Autodesk Fusion 360 part; units mm, degrees
(part 17 of 20)
  spline S293 degree 3 poles (21.9659, -337.034) (21.9695, -336.7657) (21.976, -336.2825) (22.0953, -335.8147) (22.1484, -335.6066) knots 0 0 0 0 0.080152 0.144341 0.144341 0.144341 0.144341
  spline S294 degree 3 poles (22.1484, -335.6066) (22.213, -335.4398) (22.3355, -335.1233) (22.5766, -334.8853) (22.6906, -334.7727) knots 0 0 0 0 0.052977 0.10048 0.10048 0.10048 0.10048
  spline S295 degree 3 poles (22.6906, -334.7727) (22.822, -334.6872) (23.0969, -334.5083) (23.4249, -334.4893) (23.5961, -334.4794) knots 0 0 0 0 0.046203 0.096661 0.096661 0.096661 0.096661
  spline S296 degree 3 poles (23.5961, -334.4794) (23.7239, -334.485) (23.9694, -334.4957) (24.1943, -334.5941) (24.3022, -334.6414) knots 0 0 0 0 0.037989 0.072993 0.072993 0.072993 0.072993
  spline S297 degree 3 poles (24.3022, -334.6414) (24.3994, -334.7021) (24.5968, -334.8252) (24.7339, -335.0132) (24.8035, -335.1086) knots 0 0 0 0 0.034048 0.069103 0.069103 0.069103 0.069103
  spline S298 degree 3 poles (24.8035, -335.1086) (24.8668, -335.2196) (25.0009, -335.4545) (25.0749, -335.7148) (25.1139, -335.8521) knots 0 0 0 0 0.038176 0.080832 0.080832 0.080832 0.080832
  spline S299 degree 3 poles (25.1139, -335.8521) (25.1466, -336.0232) (25.2212, -336.4133) (25.2246, -336.8107) (25.2265, -337.0339) knots 0 0 0 0 0.052146 0.118926 0.118926 0.118926 0.118926
  spline S300 degree 3 poles (25.2265, -337.0339) (25.2229, -337.3005) (25.2163, -337.7813) (25.0983, -338.247) (25.0458, -338.4545) knots 0 0 0 0 0.079639 0.143634 0.143634 0.143634 0.143634
  spline S301 degree 3 poles (25.0458, -338.4545) (24.9816, -338.6214) (24.8598, -338.9384) (24.6191, -339.1771) (24.5052, -339.2901) knots 0 0 0 0 0.052961 0.100531 0.100531 0.100531 0.100531
  spline S302 degree 3 poles (24.5052, -339.2901) (24.3736, -339.3761) (24.0979, -339.5562) (23.7684, -339.5752) (23.5963, -339.5851) knots 0 0 0 0 0.046339 0.097057 0.097057 0.097057 0.097057
  spline S303 degree 3 poles (23.5963, -339.5851) (23.37, -339.5658) (22.9288, -339.5281) (22.6139, -339.2179) (22.4605, -339.0667) knots 0 0 0 0 0.065835 0.128409 0.128409 0.128409 0.128409
  spline S304 degree 3 poles (22.4605, -339.0667) (22.3171, -338.7986) (21.9794, -338.1676) (21.9709, -337.4479) (21.9659, -337.034) knots 0 0 0 0 0.090022 0.211899 0.211899 0.211899 0.211899
  line L400 (28.3848, -338.173) -> (28.9885, -338.2514)
  spline S305 degree 3 poles (28.9885, -338.2514) (28.9458, -338.4453) (28.864, -338.8171) (28.6056, -339.0954) (28.482, -339.2286) knots 0 0 0 0 0.058356 0.111856 0.111856 0.111856 0.111856
  spline S306 degree 3 poles (28.482, -339.2286) (28.3359, -339.3315) (28.0358, -339.543) (27.6692, -339.5685) (27.481, -339.5816) knots 0 0 0 0 0.052559 0.107965 0.107965 0.107965 0.107965
  spline S307 degree 3 poles (27.481, -339.5816) (27.2479, -339.5641) (26.7963, -339.5302) (26.4521, -339.2373) (26.2856, -339.0956) knots 0 0 0 0 0.068154 0.132052 0.132052 0.132052 0.132052
  spline S308 degree 3 poles (26.2856, -339.0956) (26.154, -338.9049) (25.8661, -338.4875) (25.8451, -337.9787) (25.8336, -337.7024) knots 0 0 0 0 0.068157 0.149141 0.149141 0.149141 0.149141
  spline S309 degree 3 poles (25.8336, -337.7024) (25.8399, -337.5171) (25.8519, -337.1646) (25.9713, -336.8331) (26.028, -336.6758) knots 0 0 0 0 0.055211 0.105055 0.105055 0.105055 0.105055
  spline S310 degree 3 poles (26.028, -336.6758) (26.1002, -336.5389) (26.2424, -336.2693) (26.4952, -336.0994) (26.6197, -336.0158) knots 0 0 0 0 0.04564 0.089884 0.089884 0.089884 0.089884
  spline S311 degree 3 poles (26.6197, -336.0158) (26.7556, -335.9516) (27.0295, -335.8223) (27.332, -335.8047) (27.4843, -335.7958) knots 0 0 0 0 0.044643 0.089956 0.089956 0.089956 0.089956
  spline S312 degree 3 poles (27.4843, -335.7958) (27.668, -335.8052) (28.0159, -335.8229) (28.3105, -336.0072) (28.4495, -336.0942) knots 0 0 0 0 0.054149 0.102527 0.102527 0.102527 0.102527
  spline S313 degree 3 poles (28.4495, -336.0942) (28.564, -336.2077) (28.8031, -336.4447) (28.8868, -336.7715) (28.9305, -336.9417) knots 0 0 0 0 0.047449 0.099081 0.099081 0.099081 0.099081
  line L401 (28.9305, -336.9417) -> (28.3336, -337.0338)
  spline S314 degree 3 poles (28.3336, -337.0338) (28.3027, -336.9224) (28.2453, -336.715) (28.0993, -336.5576) (28.0317, -336.4847) knots 0 0 0 0 0.034086 0.063475 0.063475 0.063475 0.063475
  spline S315 degree 3 poles (28.0317, -336.4847) (27.9547, -336.431) (27.7974, -336.3213) (27.606, -336.3076) (27.5082, -336.3006) knots 0 0 0 0 0.027619 0.056426 0.056426 0.056426 0.056426
  spline S316 degree 3 poles (27.5082, -336.3006) (27.3615, -336.3136) (27.0724, -336.3393) (26.8594, -336.5361) (26.7545, -336.6331) knots 0 0 0 0 0.04285 0.084486 0.084486 0.084486 0.084486
  spline S317 degree 3 poles (26.7545, -336.6331) (26.6703, -336.7727) (26.4764, -337.0942) (26.4688, -337.4717) (26.4646, -337.6853) knots 0 0 0 0 0.048123 0.11083 0.11083 0.11083 0.11083
  spline S318 degree 3 poles (26.4646, -337.6853) (26.4682, -337.9011) (26.4745, -338.2798) (26.6631, -338.6058) (26.7443, -338.746) knots 0 0 0 0 0.063398 0.111295 0.111295 0.111295 0.111295
  spline S319 degree 3 poles (26.7443, -338.746) (26.8454, -338.8425) (27.05, -339.0376) (27.3317, -339.0637) (27.4742, -339.0768) knots 0 0 0 0 0.040675 0.082263 0.082263 0.082263 0.082263
  spline S320 degree 3 poles (27.4742, -339.0768) (27.5886, -339.0686) (27.8114, -339.0526) (27.9906, -338.9198) (28.0778, -338.8551) knots 0 0 0 0 0.033628 0.065508 0.065508 0.065508 0.065508
  spline S321 degree 3 poles (28.0778, -338.8551) (28.1519, -338.7651) (28.3154, -338.5665) (28.3602, -338.3121) (28.3848, -338.173) knots 0 0 0 0 0.034396 0.07593 0.07593 0.07593 0.07593
  line L402 (21.9646, -288.1562) -> (22.6093, -288.1016)
  spline S322 degree 3 poles (22.6093, -288.1016) (22.637, -288.2449) (22.6882, -288.5098) (22.862, -288.715) (22.9418, -288.8093) knots 0 0 0 0 0.042908 0.079365 0.079365 0.079365 0.079365
  spline S323 degree 3 poles (22.9418, -288.8093) (23.034, -288.8785) (23.2206, -289.0184) (23.4533, -289.037) (23.5711, -289.0464) knots 0 0 0 0 0.033826 0.068485 0.068485 0.068485 0.068485
  spline S324 degree 3 poles (23.5711, -289.0464) (23.7135, -289.0321) (24.0003, -289.0033) (24.2139, -288.8096) (24.3214, -288.7121) knots 0 0 0 0 0.041772 0.0841 0.0841 0.0841 0.0841
  spline S325 degree 3 poles (24.3214, -288.7121) (24.4109, -288.5871) (24.6001, -288.3226) (24.6186, -287.997) (24.6284, -287.8254) knots 0 0 0 0 0.045186 0.095569 0.095569 0.095569 0.095569
  spline S326 degree 3 poles (24.6284, -287.8254) (24.6193, -287.663) (24.6022, -287.3567) (24.4193, -287.1117) (24.3333, -286.9966) knots 0 0 0 0 0.047557 0.089725 0.089725 0.089725 0.089725
  spline S327 degree 3 poles (24.3333, -286.9966) (24.2248, -286.9081) (24.0003, -286.7248) (23.7106, -286.7039) (23.5608, -286.693) knots 0 0 0 0 0.040971 0.08482 0.08482 0.08482 0.08482
  spline S328 degree 3 poles (23.5608, -286.693) (23.4652, -286.6982) (23.2778, -286.7082) (23.1083, -286.7885) (23.0253, -286.8277) knots 0 0 0 0 0.028423 0.055689 0.055689 0.055689 0.055689
  spline S329 degree 3 poles (23.0253, -286.8277) (22.9505, -286.8753) (22.8036, -286.9685) (22.7007, -287.1086) (22.6502, -287.1773) knots 0 0 0 0 0.026342 0.051681 0.051681 0.051681 0.051681
  line L403 (22.6502, -287.1773) -> (22.0738, -287.1023)
  line L404 (22.0738, -287.1023) -> (22.5581, -284.5341)
  line L405 (22.5581, -284.5341) -> (25.0444, -284.5341)
  line L406 (25.0444, -284.5341) -> (25.0444, -285.1207)
  line L407 (25.0444, -285.1207) -> (23.0492, -285.1207)
  line L408 (23.0492, -285.1207) -> (22.7798, -286.4645)
  spline S330 degree 3 poles (22.7798, -286.4645) (22.9293, -286.373) (23.2201, -286.195) (23.5596, -286.1652) (23.7245, -286.1507) knots 0 0 0 0 0.051785 0.100763 0.100763 0.100763 0.100763
  spline S331 degree 3 poles (23.7245, -286.1507) (23.9338, -286.1691) (24.3494, -286.2056) (24.6702, -286.472) (24.8296, -286.6043) knots 0 0 0 0 0.061424 0.122014 0.122014 0.122014 0.122014
  spline S332 degree 3 poles (24.8296, -286.6043) (24.9609, -286.7698) (25.2317, -287.1111) (25.2634, -287.5465) (25.2798, -287.7708) knots 0 0 0 0 0.061868 0.12764 0.12764 0.12764 0.12764
  spline S333 degree 3 poles (25.2798, -287.7708) (25.2646, -287.9877) (25.2347, -288.4136) (24.9995, -288.7695) (24.8842, -288.944) knots 0 0 0 0 0.064036 0.125703 0.125703 0.125703 0.125703
  spline S334 degree 3 poles (24.8842, -288.944) (24.7064, -289.1211) (24.3434, -289.4828) (23.8321, -289.528) (23.5711, -289.5511) knots 0 0 0 0 0.072854 0.148822 0.148822 0.148822 0.148822
  spline S335 degree 3 poles (23.5711, -289.5511) (23.3578, -289.5384) (22.9503, -289.514) (22.6166, -289.2805) (22.4575, -289.1691) knots 0 0 0 0 0.062678 0.119794 0.119794 0.119794 0.119794
  spline S336 degree 3 poles (22.4575, -289.1691) (22.3288, -289.0288) (22.0646, -288.7404) (21.9985, -288.3543) (21.9646, -288.1562) knots 0 0 0 0 0.055877 0.114795 0.114795 0.114795 0.114795
  line L409 (28.3835, -288.1391) -> (28.9872, -288.2176)
  spline S337 degree 3 poles (28.9872, -288.2176) (28.9445, -288.4115) (28.8627, -288.7832) (28.6043, -289.0616) (28.4807, -289.1947) knots 0 0 0 0 0.058356 0.111856 0.111856 0.111856 0.111856
  spline S338 degree 3 poles (28.4807, -289.1947) (28.3346, -289.2977) (28.0345, -289.5091) (27.6678, -289.5346) (27.4797, -289.5477) knots 0 0 0 0 0.052559 0.107965 0.107965 0.107965 0.107965
  spline S339 degree 3 poles (27.4797, -289.5477) (27.2466, -289.5302) (26.795, -289.4963) (26.4508, -289.2034) (26.2842, -289.0617) knots 0 0 0 0 0.068154 0.132052 0.132052 0.132052 0.132052
  spline S340 degree 3 poles (26.2842, -289.0617) (26.1527, -288.871) (25.8648, -288.4536) (25.8437, -287.9448) (25.8323, -287.6685) knots 0 0 0 0 0.068157 0.149141 0.149141 0.149141 0.149141
  spline S341 degree 3 poles (25.8323, -287.6685) (25.8386, -287.4832) (25.8506, -287.1307) (25.9701, -286.7992) (26.0267, -286.6419) knots 0 0 0 0 0.055211 0.105055 0.105055 0.105055 0.105055
  spline S342 degree 3 poles (26.0267, -286.6419) (26.0989, -286.505) (26.2411, -286.2353) (26.494, -286.0655) (26.6185, -285.9819) knots 0 0 0 0 0.04564 0.089884 0.089884 0.089884 0.089884
  spline S343 degree 3 poles (26.6185, -285.9819) (26.7544, -285.9177) (27.0283, -285.7884) (27.3307, -285.7708) (27.4831, -285.7619) knots 0 0 0 0 0.044643 0.089955 0.089955 0.089955 0.089955
  spline S344 degree 3 poles (27.4831, -285.7619) (27.6668, -285.7713) (28.0147, -285.7891) (28.3093, -285.9734) (28.4483, -286.0603) knots 0 0 0 0 0.054149 0.102527 0.102527 0.102527 0.102527
  spline S345 degree 3 poles (28.4483, -286.0603) (28.5627, -286.1738) (28.8018, -286.4109) (28.8855, -286.7376) (28.9292, -286.9079) knots 0 0 0 0 0.047449 0.099081 0.099081 0.099081 0.099081
  line L410 (28.9292, -286.9079) -> (28.3323, -287)
  spline S346 degree 3 poles (28.3323, -287) (28.3014, -286.8886) (28.244, -286.6811) (28.098, -286.5237) (28.0305, -286.4509) knots 0 0 0 0 0.034086 0.063475 0.063475 0.063475 0.063475
  spline S347 degree 3 poles (28.0305, -286.4509) (27.9535, -286.3971) (27.7962, -286.2874) (27.6047, -286.2737) (27.5069, -286.2667) knots 0 0 0 0 0.027619 0.056426 0.056426 0.056426 0.056426
  spline S348 degree 3 poles (27.5069, -286.2667) (27.3603, -286.2797) (27.0711, -286.3054) (26.8581, -286.5022) (26.7532, -286.5992) knots 0 0 0 0 0.04285 0.084486 0.084486 0.084486 0.084486
  spline S349 degree 3 poles (26.7532, -286.5992) (26.669, -286.7388) (26.4751, -287.0603) (26.4676, -287.4378) (26.4633, -287.6514) knots 0 0 0 0 0.048123 0.11083 0.11083 0.11083 0.11083
  spline S350 degree 3 poles (26.4633, -287.6514) (26.4669, -287.8672) (26.4732, -288.2459) (26.6618, -288.5718) (26.743, -288.7121) knots 0 0 0 0 0.063398 0.111295 0.111295 0.111295 0.111295
  spline S351 degree 3 poles (26.743, -288.7121) (26.8441, -288.8086) (27.0487, -289.0037) (27.3304, -289.0298) (27.4728, -289.0429) knots 0 0 0 0 0.040675 0.082263 0.082263 0.082263 0.082263
  spline S352 degree 3 poles (27.4728, -289.0429) (27.5872, -289.0347) (27.8101, -289.0187) (27.9893, -288.8859) (28.0765, -288.8213) knots 0 0 0 0 0.033628 0.065508 0.065508 0.065508 0.065508
  spline S353 degree 3 poles (28.0765, -288.8213) (28.1506, -288.7313) (28.314, -288.5326) (28.3589, -288.2783) (28.3835, -288.1391) knots 0 0 0 0 0.034395 0.07593 0.07593 0.07593 0.07593
  spline S354 degree 3 poles (21.9779, -237.0342) (21.9815, -236.7658) (21.988, -236.2826) (22.1073, -235.8148) (22.1603, -235.6068) knots 0 0 0 0 0.080152 0.144341 0.144341 0.144341 0.144341
  spline S355 degree 3 poles (22.1603, -235.6068) (22.225, -235.4399) (22.3475, -235.1235) (22.5886, -234.8854) (22.7026, -234.7729) knots 0 0 0 0 0.052977 0.10048 0.10048 0.10048 0.10048
  spline S356 degree 3 poles (22.7026, -234.7729) (22.834, -234.6874) (23.1089, -234.5085) (23.4369, -234.4895) (23.6082, -234.4796) knots 0 0 0 0 0.046203 0.096661 0.096661 0.096661 0.096661
  spline S357 degree 3 poles (23.6082, -234.4796) (23.7359, -234.4852) (23.9814, -234.4959) (24.2063, -234.5944) (24.3142, -234.6416) knots 0 0 0 0 0.037989 0.072993 0.072993 0.072993 0.072993
  spline S358 degree 3 poles (24.3142, -234.6416) (24.4114, -234.7023) (24.6088, -234.8255) (24.7459, -235.0135) (24.8155, -235.1089) knots 0 0 0 0 0.034048 0.069103 0.069103 0.069103 0.069103
  spline S359 degree 3 poles (24.8155, -235.1089) (24.8788, -235.2198) (25.0128, -235.4547) (25.0868, -235.715) (25.1259, -235.8524) knots 0 0 0 0 0.038176 0.080832 0.080832 0.080832 0.080832
  spline S360 degree 3 poles (25.1259, -235.8524) (25.1586, -236.0234) (25.2332, -236.4136) (25.2365, -236.811) (25.2384, -237.0342) knots 0 0 0 0 0.052146 0.118926 0.118926 0.118926 0.118926
  spline S361 degree 3 poles (25.2384, -237.0342) (25.2348, -237.3008) (25.2282, -237.7816) (25.1102, -238.2472) (25.0577, -238.4547) knots 0 0 0 0 0.079639 0.143634 0.143634 0.143634 0.143634
  spline S362 degree 3 poles (25.0577, -238.4547) (24.9935, -238.6217) (24.8716, -238.9386) (24.631, -239.1773) (24.5171, -239.2903) knots 0 0 0 0 0.052961 0.100531 0.100531 0.100531 0.100531
  spline S363 degree 3 poles (24.5171, -239.2903) (24.3854, -239.3763) (24.1097, -239.5564) (23.7803, -239.5754) (23.6081, -239.5853) knots 0 0 0 0 0.046338 0.097057 0.097057 0.097057 0.097057
  spline S364 degree 3 poles (23.6081, -239.5853) (23.3819, -239.566) (22.9406, -239.5283) (22.6258, -239.2181) (22.4724, -239.0669) knots 0 0 0 0 0.065835 0.128409 0.128409 0.128409 0.128409
  spline S365 degree 3 poles (22.4724, -239.0669) (22.329, -238.7988) (21.9913, -238.1678) (21.9828, -237.4481) (21.9779, -237.0342) knots 0 0 0 0 0.090022 0.211899 0.211899 0.211899 0.211899
  line L411 (28.3967, -238.1734) -> (29.0004, -238.2518)
  spline S366 degree 3 poles (29.0004, -238.2518) (28.9577, -238.4457) (28.8759, -238.8174) (28.6175, -239.0958) (28.4939, -239.229) knots 0 0 0 0 0.058356 0.111856 0.111856 0.111856 0.111856
  spline S367 degree 3 poles (28.4939, -239.229) (28.3478, -239.3319) (28.0477, -239.5433) (27.681, -239.5689) (27.4928, -239.5819) knots 0 0 0 0 0.052559 0.107965 0.107965 0.107965 0.107965
  spline S368 degree 3 poles (27.4928, -239.5819) (27.2598, -239.5644) (26.8082, -239.5305) (26.464, -239.2376) (26.2974, -239.0959) knots 0 0 0 0 0.068154 0.132052 0.132052 0.132052 0.132052
  spline S369 degree 3 poles (26.2974, -239.0959) (26.1659, -238.9052) (25.878, -238.4878) (25.857, -237.979) (25.8455, -237.7027) knots 0 0 0 0 0.068157 0.149141 0.149141 0.149141 0.149141
  spline S370 degree 3 poles (25.8455, -237.7027) (25.8518, -237.5174) (25.8638, -237.1649) (25.9833, -236.8334) (26.0399, -236.6761) knots 0 0 0 0 0.055211 0.105055 0.105055 0.105055 0.105055
  spline S371 degree 3 poles (26.0399, -236.6761) (26.1121, -236.5392) (26.2543, -236.2696) (26.5072, -236.0997) (26.6317, -236.0161) knots 0 0 0 0 0.04564 0.089884 0.089884 0.089884 0.089884
  spline S372 degree 3 poles (26.6317, -236.0161) (26.7676, -235.952) (27.0415, -235.8227) (27.3439, -235.805) (27.4963, -235.7961) knots 0 0 0 0 0.044643 0.089955 0.089955 0.089955 0.089955
  spline S373 degree 3 poles (27.4963, -235.7961) (27.68, -235.8055) (28.0279, -235.8233) (28.3225, -236.0076) (28.4615, -236.0946) knots 0 0 0 0 0.054149 0.102527 0.102527 0.102527 0.102527
  spline S374 degree 3 poles (28.4615, -236.0946) (28.576, -236.2081) (28.815, -236.4451) (28.8987, -236.7719) (28.9424, -236.9421) knots 0 0 0 0 0.047449 0.099081 0.099081 0.099081 0.099081
  line L412 (28.9424, -236.9421) -> (28.3455, -237.0342)
  spline S375 degree 3 poles (28.3455, -237.0342) (28.3147, -236.9228) (28.2572, -236.7154) (28.1113, -236.558) (28.0437, -236.4851) knots 0 0 0 0 0.034086 0.063475 0.063475 0.063475 0.063475
  spline S376 degree 3 poles (28.0437, -236.4851) (27.9667, -236.4314) (27.8094, -236.3216) (27.6179, -236.3079) (27.5202, -236.3009) knots 0 0 0 0 0.027619 0.056426 0.056426 0.056426 0.056426
  spline S377 degree 3 poles (27.5202, -236.3009) (27.3735, -236.3139) (27.0844, -236.3397) (26.8714, -236.5365) (26.7664, -236.6334) knots 0 0 0 0 0.04285 0.084486 0.084486 0.084486 0.084486
  spline S378 degree 3 poles (26.7664, -236.6334) (26.6822, -236.773) (26.4883, -237.0945) (26.4808, -237.472) (26.4765, -237.6856) knots 0 0 0 0 0.048123 0.11083 0.11083 0.11083 0.11083
  spline S379 degree 3 poles (26.4765, -237.6856) (26.4801, -237.9014) (26.4864, -238.2801) (26.675, -238.6061) (26.7562, -238.7463) knots 0 0 0 0 0.063398 0.111295 0.111295 0.111295 0.111295
  spline S380 degree 3 poles (26.7562, -238.7463) (26.8573, -238.8428) (27.0619, -239.038) (27.3436, -239.064) (27.486, -239.0772) knots 0 0 0 0 0.040675 0.082263 0.082263 0.082263 0.082263
  spline S381 degree 3 poles (27.486, -239.0772) (27.6004, -239.069) (27.8233, -239.053) (28.0025, -238.9201) (28.0897, -238.8555) knots 0 0 0 0 0.033628 0.065508 0.065508 0.065508 0.065508
  spline S382 degree 3 poles (28.0897, -238.8555) (28.1638, -238.7655) (28.3272, -238.5669) (28.3721, -238.3125) (28.3967, -238.1734) knots 0 0 0 0 0.034396 0.07593 0.07593 0.07593 0.07593
  line L413 (21.9782, -188.1903) -> (22.6228, -188.1357)
  spline S383 degree 3 poles (22.6228, -188.1357) (22.6505, -188.279) (22.7018, -188.5439) (22.8755, -188.7492) (22.9553, -188.8435) knots 0 0 0 0 0.042908 0.079365 0.079365 0.079365 0.079365
  spline S384 degree 3 poles (22.9553, -188.8435) (23.0475, -188.9126) (23.2341, -189.0526) (23.4668, -189.0711) (23.5846, -189.0805) knots 0 0 0 0 0.033826 0.068485 0.068485 0.068485 0.068485
  spline S385 degree 3 poles (23.5846, -189.0805) (23.727, -189.0662) (24.0138, -189.0374) (24.2274, -188.8437) (24.3349, -188.7462) knots 0 0 0 0 0.041772 0.0841 0.0841 0.0841 0.0841
  spline S386 degree 3 poles (24.3349, -188.7462) (24.4244, -188.6212) (24.6136, -188.3567) (24.6321, -188.0311) (24.6419, -187.8595) knots 0 0 0 0 0.045186 0.095569 0.095569 0.095569 0.095569
  spline S387 degree 3 poles (24.6419, -187.8595) (24.6328, -187.6971) (24.6157, -187.3908) (24.4328, -187.1458) (24.3469, -187.0307) knots 0 0 0 0 0.047557 0.089725 0.089725 0.089725 0.089725
  spline S388 degree 3 poles (24.3469, -187.0307) (24.2384, -186.9422) (24.0138, -186.759) (23.7241, -186.738) (23.5744, -186.7271) knots 0 0 0 0 0.040971 0.08482 0.08482 0.08482 0.08482
  spline S389 degree 3 poles (23.5744, -186.7271) (23.4787, -186.7323) (23.2914, -186.7423) (23.1219, -186.8226) (23.0389, -186.8619) knots 0 0 0 0 0.028423 0.055689 0.055689 0.055689 0.055689
  spline S390 degree 3 poles (23.0389, -186.8619) (22.964, -186.9094) (22.8172, -187.0026) (22.7142, -187.1428) (22.6637, -187.2115) knots 0 0 0 0 0.026342 0.051681 0.051681 0.051681 0.051681
  line L414 (22.6637, -187.2115) -> (22.0873, -187.1364)
  line L415 (22.0873, -187.1364) -> (22.5716, -184.5682)
  line L416 (22.5716, -184.5682) -> (25.058, -184.5682)
  line L417 (25.058, -184.5682) -> (25.058, -185.1548)
  line L418 (25.058, -185.1548) -> (23.0628, -185.1548)
  line L419 (23.0628, -185.1548) -> (22.7933, -186.4986)
  spline S391 degree 3 poles (22.7933, -186.4986) (22.9428, -186.4071) (23.2337, -186.2291) (23.5731, -186.1993) (23.7381, -186.1849) knots 0 0 0 0 0.051785 0.100763 0.100763 0.100763 0.100763
  spline S392 degree 3 poles (23.7381, -186.1849) (23.9473, -186.2032) (24.3629, -186.2397) (24.6838, -186.5062) (24.8431, -186.6385) knots 0 0 0 0 0.061424 0.122014 0.122014 0.122014 0.122014
  spline S393 degree 3 poles (24.8431, -186.6385) (24.9744, -186.8039) (25.2452, -187.1452) (25.277, -187.5806) (25.2933, -187.8049) knots 0 0 0 0 0.061868 0.12764 0.12764 0.12764 0.12764
  spline S394 degree 3 poles (25.2933, -187.8049) (25.2781, -188.0219) (25.2483, -188.4477) (25.0131, -188.8036) (24.8977, -188.9782) knots 0 0 0 0 0.064036 0.125703 0.125703 0.125703 0.125703
  spline S395 degree 3 poles (24.8977, -188.9782) (24.72, -189.1552) (24.3569, -189.5169) (23.8456, -189.5622) (23.5846, -189.5853) knots 0 0 0 0 0.072854 0.148822 0.148822 0.148822 0.148822
  spline S396 degree 3 poles (23.5846, -189.5853) (23.3714, -189.5725) (22.9638, -189.5482) (22.6301, -189.3146) (22.471, -189.2033) knots 0 0 0 0 0.062678 0.119794 0.119794 0.119794 0.119794
  spline S397 degree 3 poles (22.471, -189.2033) (22.3424, -189.0629) (22.0781, -188.7746) (22.0121, -188.3885) (21.9782, -188.1903) knots 0 0 0 0 0.055877 0.114795 0.114795 0.114795 0.114795
  line L420 (28.397, -188.1733) -> (29.0007, -188.2517)
  spline S398 degree 3 poles (29.0007, -188.2517) (28.958, -188.4456) (28.8762, -188.8173) (28.6178, -189.0957) (28.4942, -189.2289) knots 0 0 0 0 0.058356 0.111856 0.111856 0.111856 0.111856
  spline S399 degree 3 poles (28.4942, -189.2289) (28.3481, -189.3318) (28.048, -189.5432) (27.6814, -189.5688) (27.4932, -189.5819) knots 0 0 0 0 0.052559 0.107965 0.107965 0.107965 0.107965
  spline S400 degree 3 poles (27.4932, -189.5819) (27.2601, -189.5643) (26.8085, -189.5304) (26.4643, -189.2376) (26.2978, -189.0958) knots 0 0 0 0 0.068154 0.132052 0.132052 0.132052 0.132052
  spline S401 degree 3 poles (26.2978, -189.0958) (26.1662, -188.9051) (25.8783, -188.4877) (25.8573, -187.9789) (25.8458, -187.7026) knots 0 0 0 0 0.068157 0.149141 0.149141 0.149141 0.149141
  spline S402 degree 3 poles (25.8458, -187.7026) (25.8522, -187.5173) (25.8642, -187.1649) (25.9836, -186.8333) (26.0403, -186.676) knots 0 0 0 0 0.055211 0.105055 0.105055 0.105055 0.105055
  spline S403 degree 3 poles (26.0403, -186.676) (26.1125, -186.5391) (26.2546, -186.2695) (26.5075, -186.0996) (26.632, -186.016) knots 0 0 0 0 0.04564 0.089884 0.089884 0.089884 0.089884
  spline S404 degree 3 poles (26.632, -186.016) (26.7679, -185.9519) (27.0418, -185.8226) (27.3443, -185.8049) (27.4966, -185.796) knots 0 0 0 0 0.044643 0.089955 0.089955 0.089955 0.089955
  spline S405 degree 3 poles (27.4966, -185.796) (27.6803, -185.8054) (28.0282, -185.8232) (28.3228, -186.0075) (28.4618, -186.0945) knots 0 0 0 0 0.054149 0.102527 0.102527 0.102527 0.102527
  spline S406 degree 3 poles (28.4618, -186.0945) (28.5763, -186.208) (28.8153, -186.445) (28.8991, -186.7717) (28.9427, -186.942) knots 0 0 0 0 0.047449 0.099081 0.099081 0.099081 0.099081
  line L421 (28.9427, -186.942) -> (28.3458, -187.0341)
  spline S407 degree 3 poles (28.3458, -187.0341) (28.315, -186.9227) (28.2575, -186.7153) (28.1116, -186.5579) (28.044, -186.485) knots 0 0 0 0 0.034086 0.063475 0.063475 0.063475 0.063475
  spline S408 degree 3 poles (28.044, -186.485) (27.967, -186.4313) (27.8097, -186.3216) (27.6182, -186.3078) (27.5205, -186.3008) knots 0 0 0 0 0.027619 0.056426 0.056426 0.056426 0.056426
  spline S409 degree 3 poles (27.5205, -186.3008) (27.3738, -186.3139) (27.0847, -186.3396) (26.8717, -186.5364) (26.7667, -186.6334) knots 0 0 0 0 0.04285 0.084486 0.084486 0.084486 0.084486
  spline S410 degree 3 poles (26.7667, -186.6334) (26.6825, -186.7729) (26.4886, -187.0944) (26.4811, -187.4719) (26.4768, -187.6855) knots 0 0 0 0 0.048123 0.11083 0.11083 0.11083 0.11083
  spline S411 degree 3 poles (26.4768, -187.6855) (26.4804, -187.9013) (26.4867, -188.28) (26.6753, -188.606) (26.7565, -188.7462) knots 0 0 0 0 0.063398 0.111295 0.111295 0.111295 0.111295
  spline S412 degree 3 poles (26.7565, -188.7462) (26.8576, -188.8427) (27.0622, -189.0379) (27.3439, -189.0639) (27.4864, -189.0771) knots 0 0 0 0 0.040675 0.082263 0.082263 0.082263 0.082263
  spline S413 degree 3 poles (27.4864, -189.0771) (27.6008, -189.0689) (27.8236, -189.0529) (28.0028, -188.92) (28.09, -188.8554) knots 0 0 0 0 0.033628 0.065508 0.065508 0.065508 0.065508
  spline S414 degree 3 poles (28.09, -188.8554) (28.1641, -188.7654) (28.3276, -188.5668) (28.3725, -188.3124) (28.397, -188.1733) knots 0 0 0 0 0.034396 0.07593 0.07593 0.07593 0.07593
  spline S415 degree 3 poles (21.944, -137.0341) (21.9477, -136.7658) (21.9542, -136.2826) (22.0735, -135.8148) (22.1265, -135.6068) knots 0 0 0 0 0.080152 0.144341 0.144341 0.144341 0.144341
  spline S416 degree 3 poles (22.1265, -135.6068) (22.1911, -135.4399) (22.3137, -135.1234) (22.5548, -134.8854) (22.6688, -134.7729) knots 0 0 0 0 0.052977 0.10048 0.10048 0.10048 0.10048
  spline S417 degree 3 poles (22.6688, -134.7729) (22.8002, -134.6874) (23.0751, -134.5085) (23.4031, -134.4895) (23.5743, -134.4795) knots 0 0 0 0 0.046203 0.096661 0.096661 0.096661 0.096661
  spline S418 degree 3 poles (23.5743, -134.4795) (23.7021, -134.4851) (23.9476, -134.4958) (24.1725, -134.5943) (24.2803, -134.6415) knots 0 0 0 0 0.037989 0.072993 0.072993 0.072993 0.072993
  spline S419 degree 3 poles (24.2803, -134.6415) (24.3776, -134.7022) (24.5749, -134.8254) (24.7121, -135.0134) (24.7817, -135.1088) knots 0 0 0 0 0.034048 0.069103 0.069103 0.069103 0.069103
  spline S420 degree 3 poles (24.7817, -135.1088) (24.845, -135.2198) (24.979, -135.4547) (25.053, -135.715) (25.0921, -135.8523) knots 0 0 0 0 0.038176 0.080832 0.080832 0.080832 0.080832
  spline S421 degree 3 poles (25.0921, -135.8523) (25.1248, -136.0234) (25.1994, -136.4135) (25.2027, -136.8109) (25.2046, -137.0341) knots 0 0 0 0 0.052146 0.118926 0.118926 0.118926 0.118926
  spline S422 degree 3 poles (25.2046, -137.0341) (25.201, -137.3007) (25.1944, -137.7815) (25.0764, -138.2472) (25.0239, -138.4546) knots 0 0 0 0 0.079639 0.143634 0.143634 0.143634 0.143634
  spline S423 degree 3 poles (25.0239, -138.4546) (24.9597, -138.6216) (24.8378, -138.9385) (24.5972, -139.1773) (24.4833, -139.2903) knots 0 0 0 0 0.052961 0.100531 0.100531 0.100531 0.100531
  spline S424 degree 3 poles (24.4833, -139.2903) (24.3516, -139.3763) (24.0759, -139.5564) (23.7465, -139.5754) (23.5743, -139.5853) knots 0 0 0 0 0.046338 0.097057 0.097057 0.097057 0.097057
  spline S425 degree 3 poles (23.5743, -139.5853) (23.3481, -139.566) (22.9068, -139.5283) (22.592, -139.218) (22.4386, -139.0669) knots 0 0 0 0 0.065835 0.128409 0.128409 0.128409 0.128409
  spline S426 degree 3 poles (22.4386, -139.0669) (22.2952, -138.7988) (21.9575, -138.1677) (21.949, -137.448) (21.944, -137.0341) knots 0 0 0 0 0.090022 0.211899 0.211899 0.211899 0.211899
  line L422 (28.3629, -138.1733) -> (28.9666, -138.2517)
  spline S427 degree 3 poles (28.9666, -138.2517) (28.9239, -138.4456) (28.8421, -138.8173) (28.5837, -139.0957) (28.4601, -139.2289) knots 0 0 0 0 0.058356 0.111856 0.111856 0.111856 0.111856
  spline S428 degree 3 poles (28.4601, -139.2289) (28.314, -139.3318) (28.0139, -139.5433) (27.6472, -139.5688) (27.4591, -139.5819) knots 0 0 0 0 0.052559 0.107965 0.107965 0.107965 0.107965
  spline S429 degree 3 poles (27.4591, -139.5819) (27.226, -139.5644) (26.7744, -139.5304) (26.4302, -139.2376) (26.2636, -139.0958) knots 0 0 0 0 0.068154 0.132052 0.132052 0.132052 0.132052
  spline S430 degree 3 poles (26.2636, -139.0958) (26.1321, -138.9051) (25.8442, -138.4877) (25.8232, -137.9789) (25.8117, -137.7026) knots 0 0 0 0 0.068157 0.149141 0.149141 0.149141 0.149141
  spline S431 degree 3 poles (25.8117, -137.7026) (25.818, -137.5173) (25.83, -137.1649) (25.9495, -136.8333) (26.0061, -136.676) knots 0 0 0 0 0.055211 0.105055 0.105055 0.105055 0.105055
  spline S432 degree 3 poles (26.0061, -136.676) (26.0783, -136.5391) (26.2205, -136.2695) (26.4734, -136.0996) (26.5979, -136.016) knots 0 0 0 0 0.04564 0.089884 0.089884 0.089884 0.089884
  spline S433 degree 3 poles (26.5979, -136.016) (26.7338, -135.9519) (27.0077, -135.8226) (27.3101, -135.8049) (27.4625, -135.7961) knots 0 0 0 0 0.044643 0.089955 0.089955 0.089955 0.089955
  spline S434 degree 3 poles (27.4625, -135.7961) (27.6462, -135.8054) (27.9941, -135.8232) (28.2887, -136.0075) (28.4277, -136.0945) knots 0 0 0 0 0.054149 0.102527 0.102527 0.102527 0.102527
  spline S435 degree 3 poles (28.4277, -136.0945) (28.5422, -136.208) (28.7812, -136.445) (28.8649, -136.7718) (28.9086, -136.942) knots 0 0 0 0 0.047449 0.099081 0.099081 0.099081 0.099081
  line L423 (28.9086, -136.942) -> (28.3117, -137.0341)
  spline S436 degree 3 poles (28.3117, -137.0341) (28.2809, -136.9227) (28.2234, -136.7153) (28.0774, -136.5579) (28.0099, -136.485) knots 0 0 0 0 0.034086 0.063475 0.063475 0.063475 0.063475
  spline S437 degree 3 poles (28.0099, -136.485) (27.9329, -136.4313) (27.7756, -136.3216) (27.5841, -136.3078) (27.4863, -136.3008) knots 0 0 0 0 0.027619 0.056426 0.056426 0.056426 0.056426
  spline S438 degree 3 poles (27.4863, -136.3008) (27.3397, -136.3139) (27.0505, -136.3396) (26.8376, -136.5364) (26.7326, -136.6334) knots 0 0 0 0 0.04285 0.084486 0.084486 0.084486 0.084486
  spline S439 degree 3 poles (26.7326, -136.6334) (26.6484, -136.7729) (26.4545, -137.0944) (26.447, -137.4719) (26.4427, -137.6855) knots 0 0 0 0 0.048123 0.11083 0.11083 0.11083 0.11083
  spline S440 degree 3 poles (26.4427, -137.6855) (26.4463, -137.9013) (26.4526, -138.28) (26.6412, -138.606) (26.7224, -138.7463) knots 0 0 0 0 0.063398 0.111295 0.111295 0.111295 0.111295
  spline S441 degree 3 poles (26.7224, -138.7463) (26.8235, -138.8427) (27.0281, -139.0379) (27.3098, -139.0639) (27.4522, -139.0771) knots 0 0 0 0 0.040675 0.082263 0.082263 0.082263 0.082263
  spline S442 degree 3 poles (27.4522, -139.0771) (27.5666, -139.0689) (27.7895, -139.0529) (27.9687, -138.92) (28.0559, -138.8554) knots 0 0 0 0 0.033628 0.065508 0.065508 0.065508 0.065508
  spline S443 degree 3 poles (28.0559, -138.8554) (28.13, -138.7654) (28.2934, -138.5668) (28.3383, -138.3124) (28.3629, -138.1733) knots 0 0 0 0 0.034396 0.07593 0.07593 0.07593 0.07593
  line L424 (21.9441, -88.1579) -> (22.5887, -88.1033)
  spline S444 degree 3 poles (22.5887, -88.1033) (22.6164, -88.2466) (22.6677, -88.5115) (22.8414, -88.7168) (22.9212, -88.811) knots 0 0 0 0 0.042908 0.079365 0.079365 0.079365 0.079365
  spline S445 degree 3 poles (22.9212, -88.811) (23.0134, -88.8802) (23.2, -89.0201) (23.4327, -89.0387) (23.5505, -89.0481) knots 0 0 0 0 0.033826 0.068485 0.068485 0.068485 0.068485
  spline S446 degree 3 poles (23.5505, -89.0481) (23.6929, -89.0338) (23.9797, -89.005) (24.1933, -88.8113) (24.3008, -88.7138) knots 0 0 0 0 0.041772 0.0841 0.0841 0.0841 0.0841
  spline S447 degree 3 poles (24.3008, -88.7138) (24.3903, -88.5888) (24.5795, -88.3243) (24.598, -87.9987) (24.6078, -87.8271) knots 0 0 0 0 0.045186 0.095569 0.095569 0.095569 0.095569
  spline S448 degree 3 poles (24.6078, -87.8271) (24.5987, -87.6647) (24.5816, -87.3584) (24.3987, -87.1134) (24.3128, -86.9983) knots 0 0 0 0 0.047557 0.089725 0.089725 0.089725 0.089725
  spline S449 degree 3 poles (24.3128, -86.9983) (24.2043, -86.9098) (23.9797, -86.7266) (23.69, -86.7056) (23.5403, -86.6947) knots 0 0 0 0 0.040971 0.08482 0.08482 0.08482 0.08482
  spline S450 degree 3 poles (23.5403, -86.6947) (23.4446, -86.6999) (23.2573, -86.7099) (23.0878, -86.7902) (23.0048, -86.8295) knots 0 0 0 0 0.028423 0.055689 0.055689 0.055689 0.055689
  spline S451 degree 3 poles (23.0048, -86.8295) (22.9299, -86.877) (22.7831, -86.9702) (22.6801, -87.1104) (22.6296, -87.1791) knots 0 0 0 0 0.026342 0.051681 0.051681 0.051681 0.051681
  line L425 (22.6296, -87.1791) -> (22.0532, -87.104)
  line L426 (22.0532, -87.104) -> (22.5375, -84.5358)
  line L427 (22.5375, -84.5358) -> (25.0239, -84.5358)
  line L428 (25.0239, -84.5358) -> (25.0239, -85.1224)
  line L429 (25.0239, -85.1224) -> (23.0287, -85.1224)
  line L430 (23.0287, -85.1224) -> (22.7592, -86.4662)
  spline S452 degree 3 poles (22.7592, -86.4662) (22.9087, -86.3747) (23.1996, -86.1967) (23.539, -86.1669) (23.704, -86.1524) knots 0 0 0 0 0.051785 0.100763 0.100763 0.100763 0.100763
  spline S453 degree 3 poles (23.704, -86.1524) (23.9132, -86.1708) (24.3288, -86.2073) (24.6497, -86.4738) (24.809, -86.6061) knots 0 0 0 0 0.061424 0.122014 0.122014 0.122014 0.122014
  spline S454 degree 3 poles (24.809, -86.6061) (24.9403, -86.7715) (25.2111, -87.1128) (25.2429, -87.5482) (25.2592, -87.7725) knots 0 0 0 0 0.061868 0.127641 0.127641 0.127641 0.127641
  spline S455 degree 3 poles (25.2592, -87.7725) (25.244, -87.9895) (25.2142, -88.4153) (24.979, -88.7712) (24.8636, -88.9458) knots 0 0 0 0 0.064036 0.125703 0.125703 0.125703 0.125703
  spline S456 degree 3 poles (24.8636, -88.9458) (24.6858, -89.1228) (24.3228, -89.4845) (23.8115, -89.5297) (23.5505, -89.5529) knots 0 0 0 0 0.072854 0.148822 0.148822 0.148822 0.148822
  spline S457 degree 3 poles (23.5505, -89.5529) (23.3373, -89.5401) (22.9297, -89.5158) (22.596, -89.2822) (22.4369, -89.1709) knots 0 0 0 0 0.062678 0.119794 0.119794 0.119794 0.119794
  spline S458 degree 3 poles (22.4369, -89.1709) (22.3083, -89.0305) (22.044, -88.7421) (21.978, -88.3561) (21.9441, -88.1579) knots 0 0 0 0 0.055877 0.114795 0.114795 0.114795 0.114795
  line L431 (28.3629, -88.1409) -> (28.9666, -88.2193)
  spline S459 degree 3 poles (28.9666, -88.2193) (28.9239, -88.4132) (28.8421, -88.7849) (28.5837, -89.0633) (28.4601, -89.1964) knots 0 0 0 0 0.058356 0.111856 0.111856 0.111856 0.111856
  spline S460 degree 3 poles (28.4601, -89.1964) (28.314, -89.2994) (28.0139, -89.5108) (27.6473, -89.5364) (27.4591, -89.5494) knots 0 0 0 0 0.052559 0.107965 0.107965 0.107965 0.107965
  spline S461 degree 3 poles (27.4591, -89.5494) (27.226, -89.5319) (26.7744, -89.498) (26.4302, -89.2051) (26.2636, -89.0634) knots 0 0 0 0 0.068154 0.132052 0.132052 0.132052 0.132052
  spline S462 degree 3 poles (26.2636, -89.0634) (26.1321, -88.8727) (25.8442, -88.4553) (25.8232, -87.9465) (25.8117, -87.6702) knots 0 0 0 0 0.068157 0.149141 0.149141 0.149141 0.149141
  spline S463 degree 3 poles (25.8117, -87.6702) (25.818, -87.4849) (25.8301, -87.1324) (25.9495, -86.8009) (26.0061, -86.6436) knots 0 0 0 0 0.055211 0.105055 0.105055 0.105055 0.105055
  spline S464 degree 3 poles (26.0061, -86.6436) (26.0783, -86.5067) (26.2205, -86.2371) (26.4734, -86.0672) (26.5979, -85.9836) knots 0 0 0 0 0.04564 0.089884 0.089884 0.089884 0.089884
  spline S465 degree 3 poles (26.5979, -85.9836) (26.7338, -85.9195) (27.0077, -85.7902) (27.3101, -85.7725) (27.4625, -85.7636) knots 0 0 0 0 0.044643 0.089956 0.089956 0.089956 0.089956
  spline S466 degree 3 poles (27.4625, -85.7636) (27.6462, -85.773) (27.9941, -85.7908) (28.2887, -85.9751) (28.4277, -86.0621) knots 0 0 0 0 0.054149 0.102527 0.102527 0.102527 0.102527
  spline S467 degree 3 poles (28.4277, -86.0621) (28.5422, -86.1756) (28.7812, -86.4126) (28.865, -86.7393) (28.9086, -86.9096) knots 0 0 0 0 0.047449 0.099081 0.099081 0.099081 0.099081
  line L432 (28.9086, -86.9096) -> (28.3117, -87.0017)
  spline S468 degree 3 poles (28.3117, -87.0017) (28.2809, -86.8903) (28.2234, -86.6829) (28.0775, -86.5255) (28.0099, -86.4526) knots 0 0 0 0 0.034086 0.063475 0.063475 0.063475 0.063475
  spline S469 degree 3 poles (28.0099, -86.4526) (27.9329, -86.3989) (27.7756, -86.2891) (27.5841, -86.2754) (27.4864, -86.2684) knots 0 0 0 0 0.027619 0.056426 0.056426 0.056426 0.056426
  spline S470 degree 3 poles (27.4864, -86.2684) (27.3397, -86.2815) (27.0506, -86.3072) (26.8376, -86.504) (26.7326, -86.6009) knots 0 0 0 0 0.04285 0.084486 0.084486 0.084486 0.084486
  spline S471 degree 3 poles (26.7326, -86.6009) (26.6484, -86.7405) (26.4545, -87.062) (26.447, -87.4395) (26.4427, -87.6531) knots 0 0 0 0 0.048123 0.11083 0.11083 0.11083 0.11083
  spline S472 degree 3 poles (26.4427, -87.6531) (26.4463, -87.8689) (26.4526, -88.2476) (26.6412, -88.5736) (26.7224, -88.7138) knots 0 0 0 0 0.063398 0.111295 0.111295 0.111295 0.111295
  spline S473 degree 3 poles (26.7224, -88.7138) (26.8235, -88.8103) (27.0281, -89.0055) (27.3098, -89.0315) (27.4523, -89.0447) knots 0 0 0 0 0.040675 0.082263 0.082263 0.082263 0.082263
  spline S474 degree 3 poles (27.4523, -89.0447) (27.5666, -89.0365) (27.7895, -89.0205) (27.9687, -88.8876) (28.0559, -88.823) knots 0 0 0 0 0.033628 0.065508 0.065508 0.065508 0.065508
  spline S475 degree 3 poles (28.0559, -88.823) (28.13, -88.733) (28.2935, -88.5344) (28.3383, -88.28) (28.3629, -88.1409) knots 0 0 0 0 0.034396 0.07593 0.07593 0.07593 0.07593
  spline S476 degree 3 poles (21.9679, -37.0341) (21.9715, -36.7658) (21.9781, -36.2826) (22.0973, -35.8148) (22.1504, -35.6068) knots 0 0 0 0 0.080152 0.144341 0.144341 0.144341 0.144341
  spline S477 degree 3 poles (22.1504, -35.6068) (22.215, -35.4399) (22.3376, -35.1234) (22.5787, -34.8854) (22.6927, -34.7729) knots 0 0 0 0 0.052977 0.10048 0.10048 0.10048 0.10048
  spline S478 degree 3 poles (22.6927, -34.7729) (22.8241, -34.6874) (23.0989, -34.5085) (23.427, -34.4895) (23.5982, -34.4795) knots 0 0 0 0 0.046203 0.096661 0.096661 0.096661 0.096661
  spline S479 degree 3 poles (23.5982, -34.4795) (23.726, -34.4851) (23.9715, -34.4958) (24.1964, -34.5943) (24.3042, -34.6415) knots 0 0 0 0 0.037989 0.072993 0.072993 0.072993 0.072993
  spline S480 degree 3 poles (24.3042, -34.6415) (24.4015, -34.7022) (24.5988, -34.8254) (24.736, -35.0134) (24.8056, -35.1088) knots 0 0 0 0 0.034048 0.069103 0.069103 0.069103 0.069103
  spline S481 degree 3 poles (24.8056, -35.1088) (24.8689, -35.2198) (25.0029, -35.4547) (25.0769, -35.715) (25.116, -35.8523) knots 0 0 0 0 0.038176 0.080832 0.080832 0.080832 0.080832
  spline S482 degree 3 poles (25.116, -35.8523) (25.1487, -36.0234) (25.2232, -36.4135) (25.2266, -36.8109) (25.2285, -37.0341) knots 0 0 0 0 0.052146 0.118926 0.118926 0.118926 0.118926
  spline S483 degree 3 poles (25.2285, -37.0341) (25.2249, -37.3007) (25.2183, -37.7815) (25.1003, -38.2472) (25.0477, -38.4546) knots 0 0 0 0 0.079639 0.143634 0.143634 0.143634 0.143634
  spline S484 degree 3 poles (25.0477, -38.4546) (24.9836, -38.6216) (24.8617, -38.9385) (24.621, -39.1773) (24.5072, -39.2903) knots 0 0 0 0 0.052961 0.100531 0.100531 0.100531 0.100531
  spline S485 degree 3 poles (24.5072, -39.2903) (24.3755, -39.3763) (24.0998, -39.5564) (23.7704, -39.5754) (23.5982, -39.5853) knots 0 0 0 0 0.046338 0.097057 0.097057 0.097057 0.097057
  spline S486 degree 3 poles (23.5982, -39.5853) (23.372, -39.566) (22.9307, -39.5283) (22.6159, -39.218) (22.4625, -39.0669) knots 0 0 0 0 0.065835 0.128409 0.128409 0.128409 0.128409
  spline S487 degree 3 poles (22.4625, -39.0669) (22.319, -38.7988) (21.9814, -38.1677) (21.9729, -37.448) (21.9679, -37.0341) knots 0 0 0 0 0.090022 0.211899 0.211899 0.211899 0.211899
  line L433 (28.3868, -38.1733) -> (28.9904, -38.2517)
  spline S488 degree 3 poles (28.9904, -38.2517) (28.9478, -38.4456) (28.866, -38.8173) (28.6076, -39.0957) (28.484, -39.2289) knots 0 0 0 0 0.058356 0.111856 0.111856 0.111856 0.111856
  spline S489 degree 3 poles (28.484, -39.2289) (28.3379, -39.3318) (28.0378, -39.5433) (27.6711, -39.5688) (27.4829, -39.5819) knots 0 0 0 0 0.052559 0.107965 0.107965 0.107965 0.107965
  spline S490 degree 3 poles (27.4829, -39.5819) (27.2499, -39.5644) (26.7983, -39.5304) (26.4541, -39.2376) (26.2875, -39.0958) knots 0 0 0 0 0.068154 0.132052 0.132052 0.132052 0.132052
  spline S491 degree 3 poles (26.2875, -39.0958) (26.156, -38.9051) (25.8681, -38.4877) (25.847, -37.9789) (25.8356, -37.7026) knots 0 0 0 0 0.068157 0.149141 0.149141 0.149141 0.149141
  spline S492 degree 3 poles (25.8356, -37.7026) (25.8419, -37.5174) (25.8539, -37.1649) (25.9733, -36.8333) (26.03, -36.676) knots 0 0 0 0 0.055211 0.105055 0.105055 0.105055 0.105055
  spline S493 degree 3 poles (26.03, -36.676) (26.1022, -36.5391) (26.2444, -36.2695) (26.4973, -36.0996) (26.6218, -36.016) knots 0 0 0 0 0.04564 0.089884 0.089884 0.089884 0.089884
  spline S494 degree 3 poles (26.6218, -36.016) (26.7577, -35.9519) (27.0316, -35.8226) (27.334, -35.8049) (27.4863, -35.7961) knots 0 0 0 0 0.044643 0.089955 0.089955 0.089955 0.089955
  spline S495 degree 3 poles (27.4863, -35.7961) (27.6701, -35.8054) (28.018, -35.8232) (28.3126, -36.0075) (28.4516, -36.0945) knots 0 0 0 0 0.054149 0.102527 0.102527 0.102527 0.102527
  spline S496 degree 3 poles (28.4516, -36.0945) (28.566, -36.208) (28.8051, -36.445) (28.8888, -36.7718) (28.9325, -36.942) knots 0 0 0 0 0.047449 0.099081 0.099081 0.099081 0.099081
  line L434 (28.9325, -36.942) -> (28.3356, -37.0341)
  spline S497 degree 3 poles (28.3356, -37.0341) (28.3047, -36.9227) (28.2473, -36.7153) (28.1013, -36.5579) (28.0338, -36.485) knots 0 0 0 0 0.034086 0.063475 0.063475 0.063475 0.063475
  spline S498 degree 3 poles (28.0338, -36.485) (27.9568, -36.4313) (27.7995, -36.3216) (27.608, -36.3078) (27.5102, -36.3008) knots 0 0 0 0 0.027619 0.056426 0.056426 0.056426 0.056426
  spline S499 degree 3 poles (27.5102, -36.3008) (27.3636, -36.3139) (27.0744, -36.3396) (26.8614, -36.5364) (26.7565, -36.6334) knots 0 0 0 0 0.04285 0.084486 0.084486 0.084486 0.084486
  spline S500 degree 3 poles (26.7565, -36.6334) (26.6723, -36.7729) (26.4784, -37.0944) (26.4708, -37.4719) (26.4666, -37.6855) knots 0 0 0 0 0.048123 0.11083 0.11083 0.11083 0.11083
  spline S501 degree 3 poles (26.4666, -37.6855) (26.4702, -37.9013) (26.4764, -38.28) (26.6651, -38.606) (26.7462, -38.7463) knots 0 0 0 0 0.063398 0.111295 0.111295 0.111295 0.111295
  spline S502 degree 3 poles (26.7462, -38.7463) (26.8474, -38.8427) (27.0519, -39.0379) (27.3337, -39.0639) (27.4761, -39.0771) knots 0 0 0 0 0.040675 0.082263 0.082263 0.082263 0.082263
  spline S503 degree 3 poles (27.4761, -39.0771) (27.5905, -39.0689) (27.8133, -39.0529) (27.9926, -38.92) (28.0798, -38.8554) knots 0 0 0 0 0.033628 0.065508 0.065508 0.065508 0.065508
  spline S504 degree 3 poles (28.0798, -38.8554) (28.1538, -38.7654) (28.3173, -38.5668) (28.3622, -38.3124) (28.3868, -38.1733) knots 0 0 0 0 0.034395 0.07593 0.07593 0.07593 0.07593
  line L435 (29.5157, -39.5) -> (29.5157, -35.8779)
  line L436 (29.5157, -35.8779) -> (30.0648, -35.8779)
  line L437 (30.0648, -35.8779) -> (30.0648, -36.3861)
  spline S505 degree 3 poles (30.0648, -36.3861) (30.1267, -36.3015) (30.2516, -36.131) (30.429, -36.016) (30.5184, -35.9581) knots 0 0 0 0 0.031158 0.062835 0.062835 0.062835 0.062835
  spline S506 degree 3 poles (30.5184, -35.9581) (30.6176, -35.9108) (30.8215, -35.8137) (31.0471, -35.802) (31.163, -35.7961) knots 0 0 0 0 0.032617 0.067048 0.067048 0.067048 0.067048
  spline S507 degree 3 poles (31.163, -35.7961) (31.2875, -35.8008) (31.5199, -35.8096) (31.7269, -35.9145) (31.823, -35.9632) knots 0 0 0 0 0.036859 0.068796 0.068796 0.068796 0.068796
  spline S508 degree 3 poles (31.823, -35.9632) (31.9027, -36.0249) (32.0636, -36.1496) (32.1451, -36.3362) (32.1862, -36.4304) knots 0 0 0 0 0.029725 0.060035 0.060035 0.060035 0.060035
  spline S509 degree 3 poles (32.1862, -36.4304) (32.3364, -36.2455) (32.6275, -35.8869) (33.0839, -35.8257) (33.3049, -35.7961) knots 0 0 0 0 0.068625 0.133023 0.133023 0.133023 0.133023
  spline S510 degree 3 poles (33.3049, -35.7961) (33.47, -35.8045) (33.7779, -35.8202) (34.021, -36.0076) (34.1337, -36.0945) knots 0 0 0 0 0.048244 0.08997 0.08997 0.08997 0.08997
  spline S511 degree 3 poles (34.1337, -36.0945) (34.218, -36.2168) (34.4074, -36.4917) (34.4178, -36.8274) (34.4236, -37.0137) knots 0 0 0 0 0.043695 0.098195 0.098195 0.098195 0.098195
  line L438 (34.4236, -37.0137) -> (34.4236, -39.5)
  line L439 (34.4236, -39.5) -> (33.8131, -39.5)
  line L440 (33.8131, -39.5) -> (33.8131, -37.2183)
  spline S512 degree 3 poles (33.8131, -37.2183) (33.8131, -37.1121) (33.813, -36.9328) (33.7707, -36.7588) (33.7534, -36.6879) knots 0 0 0 0 0.031711 0.053535 0.053535 0.053535 0.053535
  spline S513 degree 3 poles (33.7534, -36.6879) (33.729, -36.6363) (33.6791, -36.5309) (33.5849, -36.4621) (33.5368, -36.427) knots 0 0 0 0 0.016863 0.034394 0.034394 0.034394 0.034394
  spline S514 degree 3 poles (33.5368, -36.427) (33.4811, -36.3982) (33.3657, -36.3384) (33.2357, -36.3316) (33.1685, -36.3281) knots 0 0 0 0 0.018597 0.038532 0.038532 0.038532 0.038532
  spline S515 degree 3 poles (33.1685, -36.3281) (33.0473, -36.3379) (32.8094, -36.3572) (32.6247, -36.5081) (32.5341, -36.5822) knots 0 0 0 0 0.035532 0.069798 0.069798 0.069798 0.069798
  spline S516 degree 3 poles (32.5341, -36.5822) (32.4608, -36.6889) (32.2936, -36.9321) (32.286, -37.229) (32.2817, -37.3956) knots 0 0 0 0 0.038079 0.086792 0.086792 0.086792 0.086792
  line L441 (32.2817, -37.3956) -> (32.2817, -39.5)
  line L442 (32.2817, -39.5) -> (31.6678, -39.5)
  line L443 (31.6678, -39.5) -> (31.6678, -37.1467)
  spline S517 degree 3 poles (31.6678, -37.1467) (31.6654, -37.0246) (31.6611, -36.8078) (31.5613, -36.6164) (31.5177, -36.5328) knots 0 0 0 0 0.036008 0.063954 0.063954 0.063954 0.063954
  spline S518 degree 3 poles (31.5177, -36.5328) (31.4555, -36.4732) (31.3193, -36.3428) (31.1296, -36.3333) (31.0266, -36.3281) knots 0 0 0 0 0.025037 0.054812 0.054812 0.054812 0.054812
  spline S519 degree 3 poles (31.0266, -36.3281) (30.9418, -36.3338) (30.7724, -36.3451) (30.6224, -36.4248) (30.5474, -36.4645) knots 0 0 0 0 0.025172 0.050327 0.050327 0.050327 0.050327
  spline S520 degree 3 poles (30.5474, -36.4645) (30.4788, -36.5162) (30.3385, -36.6218) (30.2657, -36.7818) (30.2285, -36.8636) knots 0 0 0 0 0.025339 0.051812 0.051812 0.051812 0.051812
  spline S521 degree 3 poles (30.2285, -36.8636) (30.1998, -36.9699) (30.133, -37.2174) (30.1308, -37.4742) (30.1296, -37.6207) knots 0 0 0 0 0.032907 0.076633 0.076633 0.076633 0.076633
  line L444 (30.1296, -37.6207) -> (30.1296, -39.5)
  line L445 (30.1296, -39.5) -> (29.5157, -39.5)
  spline S522 degree 3 poles (19.028, -36.7885) (18.9112, -36.7401) (18.6922, -36.6493) (18.5352, -36.4722) (18.4618, -36.3895) knots 0 0 0 0 0.037333 0.070073 0.070073 0.070073 0.070073
  spline S523 degree 3 poles (18.4618, -36.3895) (18.4081, -36.2969) (18.2969, -36.1051) (18.2842, -35.8834) (18.2776, -35.7688) knots 0 0 0 0 0.031652 0.065561 0.065561 0.065561 0.065561
  spline S524 degree 3 poles (18.2776, -35.7688) (18.2938, -35.5943) (18.326, -35.2463) (18.5554, -34.9827) (18.6698, -34.8513) knots 0 0 0 0 0.05117 0.102058 0.102058 0.102058 0.102058
  spline S525 degree 3 poles (18.6698, -34.8513) (18.8165, -34.7429) (19.1259, -34.5144) (19.511, -34.4915) (19.7135, -34.4795) knots 0 0 0 0 0.053536 0.112931 0.112931 0.112931 0.112931
  spline S526 degree 3 poles (19.7135, -34.4795) (19.9176, -34.4921) (20.307, -34.5161) (20.6189, -34.749) (20.7674, -34.8598) knots 0 0 0 0 0.059849 0.114229 0.114229 0.114229 0.114229
  spline S527 degree 3 poles (20.7674, -34.8598) (20.8838, -34.9932) (21.1159, -35.2592) (21.1496, -35.6106) (21.1664, -35.7858) knots 0 0 0 0 0.051706 0.103118 0.103118 0.103118 0.103118
  spline S528 degree 3 poles (21.1664, -35.7858) (21.1597, -35.8968) (21.1464, -36.1132) (21.0372, -36.3002) (20.984, -36.3912) knots 0 0 0 0 0.032847 0.064022 0.064022 0.064022 0.064022
  spline S529 degree 3 poles (20.984, -36.3912) (20.9118, -36.4734) (20.7582, -36.6484) (20.5436, -36.74) (20.4297, -36.7885) knots 0 0 0 0 0.032377 0.06897 0.06897 0.06897 0.06897
  spline S530 degree 3 poles (20.4297, -36.7885) (20.5721, -36.8436) (20.8449, -36.9492) (21.0382, -37.1681) (21.1306, -37.2729) knots 0 0 0 0 0.045038 0.086311 0.086311 0.086311 0.086311
  spline S531 degree 3 poles (21.1306, -37.2729) (21.2007, -37.392) (21.3456, -37.6382) (21.3624, -37.9236) (21.3711, -38.0709) knots 0 0 0 0 0.040859 0.084421 0.084421 0.084421 0.084421
  spline S532 degree 3 poles (21.3711, -38.0709) (21.3526, -38.2758) (21.3157, -38.6833) (21.0498, -38.9941) (20.9175, -39.1487) knots 0 0 0 0 0.060084 0.11955 0.11955 0.11955 0.11955
  spline S533 degree 3 poles (20.9175, -39.1487) (20.7492, -39.276) (20.3968, -39.5425) (19.9547, -39.5706) (19.7237, -39.5853) knots 0 0 0 0 0.061894 0.129627 0.129627 0.129627 0.129627
  spline S534 degree 3 poles (19.7237, -39.5853) (19.4927, -39.5705) (19.0503, -39.5422) (18.6982, -39.2748) (18.53, -39.147) knots 0 0 0 0 0.067741 0.129702 0.129702 0.129702 0.129702
  spline S535 degree 3 poles (18.53, -39.147) (18.3977, -38.9908) (18.1303, -38.6749) (18.0945, -38.2624) (18.0764, -38.0539) knots 0 0 0 0 0.059851 0.120982 0.120982 0.120982 0.120982
  spline S536 degree 3 poles (18.0764, -38.0539) (18.0847, -37.9007) (18.1005, -37.6077) (18.2516, -37.3568) (18.3237, -37.237) knots 0 0 0 0 0.045232 0.08651 0.08651 0.08651 0.08651
  spline S537 degree 3 poles (18.3237, -37.237) (18.4175, -37.1354) (18.6124, -36.9242) (18.886, -36.8349) (19.028, -36.7885) knots 0 0 0 0 0.04079 0.084746 0.084746 0.084746 0.084746
  line L446 (29.4918, -89.4676) -> (29.4918, -85.8455)
  line L447 (29.4918, -85.8455) -> (30.0409, -85.8455)
  line L448 (30.0409, -85.8455) -> (30.0409, -86.3537)
  spline S538 degree 3 poles (30.0409, -86.3537) (30.1029, -86.2691) (30.2277, -86.0986) (30.4051, -85.9836) (30.4945, -85.9256) knots 0 0 0 0 0.031158 0.062835 0.062835 0.062835 0.062835
  spline S539 degree 3 poles (30.4945, -85.9256) (30.5937, -85.8784) (30.7976, -85.7813) (31.0233, -85.7696) (31.1392, -85.7636) knots 0 0 0 0 0.032617 0.067048 0.067048 0.067048 0.067048
  spline S540 degree 3 poles (31.1392, -85.7636) (31.2637, -85.7684) (31.496, -85.7772) (31.703, -85.8821) (31.7991, -85.9308) knots 0 0 0 0 0.036859 0.068796 0.068796 0.068796 0.068796
  spline S541 degree 3 poles (31.7991, -85.9308) (31.8788, -85.9925) (32.0397, -86.1172) (32.1212, -86.3038) (32.1624, -86.398) knots 0 0 0 0 0.029725 0.060035 0.060035 0.060035 0.060035